Autodesk Inventor part; units mm, degrees
(part 11 of 13)
  spline S1517 degree 3 poles (37.29, 16.1547) (37.0431, 16.1547) (36.843, 15.9546) (36.843, 15.7078) knots 0 0 0 0 1 1 1 1
  line L4777 (37.29, 16.1547) -> (37.0431, 16.1547) construction
  line L4778 (37.0431, 16.1547) -> (36.843, 15.9546) construction
  line L4779 (36.843, 15.9546) -> (36.843, 15.7078) construction
  spline S1518 degree 3 poles (36.843, 15.7078) (36.843, 15.461) (37.0431, 15.2608) (37.29, 15.2608) knots 0 0 0 0 1 1 1 1
  line L4780 (36.843, 15.7078) -> (36.843, 15.461) construction
  line L4781 (36.843, 15.461) -> (37.0431, 15.2608) construction
  line L4782 (37.0431, 15.2608) -> (37.29, 15.2608) construction
  spline S1519 degree 3 poles (37.29, 15.2608) (37.5369, 15.2608) (37.737, 15.461) (37.737, 15.7078) knots 0 0 0 0 1 1 1 1
  line L4783 (37.29, 15.2608) -> (37.5369, 15.2608) construction
  line L4784 (37.5369, 15.2608) -> (37.737, 15.461) construction
  line L4785 (37.737, 15.461) -> (37.737, 15.7078) construction
  spline S1520 degree 3 poles (35.1829, 18.2619) (35.1829, 18.5087) (34.9826, 18.7088) (34.7358, 18.7088) knots 0 0 0 0 1 1 1 1
  line L4786 (35.1829, 18.2619) -> (35.1829, 18.5087) construction
  line L4787 (35.1829, 18.5087) -> (34.9826, 18.7088) construction
  line L4788 (34.9826, 18.7088) -> (34.7358, 18.7088) construction
  spline S1521 degree 3 poles (34.7358, 18.7088) (34.4891, 18.7088) (34.289, 18.5087) (34.289, 18.2619) knots 0 0 0 0 1 1 1 1
  line L4789 (34.7358, 18.7088) -> (34.4891, 18.7088) construction
  line L4790 (34.4891, 18.7088) -> (34.289, 18.5087) construction
  line L4791 (34.289, 18.5087) -> (34.289, 18.2619) construction
  spline S1522 degree 3 poles (34.289, 18.2619) (34.289, 18.0151) (34.4891, 17.8149) (34.7358, 17.8149) knots 0 0 0 0 1 1 1 1
  line L4792 (34.289, 18.2619) -> (34.289, 18.0151) construction
  line L4793 (34.289, 18.0151) -> (34.4891, 17.8149) construction
  line L4794 (34.4891, 17.8149) -> (34.7358, 17.8149) construction
  spline S1523 degree 3 poles (34.7358, 17.8149) (34.9826, 17.8149) (35.1829, 18.0151) (35.1829, 18.2619) knots 0 0 0 0 1 1 1 1
  line L4795 (34.7358, 17.8149) -> (34.9826, 17.8149) construction
  line L4796 (34.9826, 17.8149) -> (35.1829, 18.0151) construction
  line L4797 (35.1829, 18.0151) -> (35.1829, 18.2619) construction
  spline S1524 degree 3 poles (37.737, 18.2619) (37.737, 18.5087) (37.5369, 18.7088) (37.29, 18.7088) knots 0 0 0 0 1 1 1 1
  line L4798 (37.737, 18.2619) -> (37.737, 18.5087) construction
  line L4799 (37.737, 18.5087) -> (37.5369, 18.7088) construction
  line L4800 (37.5369, 18.7088) -> (37.29, 18.7088) construction
  spline S1525 degree 3 poles (37.29, 18.7088) (37.0431, 18.7088) (36.843, 18.5087) (36.843, 18.2619) knots 0 0 0 0 1 1 1 1
  line L4801 (37.29, 18.7088) -> (37.0431, 18.7088) construction
  line L4802 (37.0431, 18.7088) -> (36.843, 18.5087) construction
  line L4803 (36.843, 18.5087) -> (36.843, 18.2619) construction
  spline S1526 degree 3 poles (36.843, 18.2619) (36.843, 18.0151) (37.0431, 17.8149) (37.29, 17.8149) knots 0 0 0 0 1 1 1 1
  line L4804 (36.843, 18.2619) -> (36.843, 18.0151) construction
  line L4805 (36.843, 18.0151) -> (37.0431, 17.8149) construction
  line L4806 (37.0431, 17.8149) -> (37.29, 17.8149) construction
  spline S1527 degree 3 poles (37.29, 17.8149) (37.5369, 17.8149) (37.737, 18.0151) (37.737, 18.2619) knots 0 0 0 0 1 1 1 1
  line L4807 (37.29, 17.8149) -> (37.5369, 17.8149) construction
  line L4808 (37.5369, 17.8149) -> (37.737, 18.0151) construction
  line L4809 (37.737, 18.0151) -> (37.737, 18.2619) construction
  spline S1528 degree 3 poles (35.1829, 20.816) (35.1829, 21.0628) (34.9826, 21.2629) (34.7358, 21.2629) knots 0 0 0 0 1 1 1 1
  line L4810 (35.1829, 20.816) -> (35.1829, 21.0628) construction
  line L4811 (35.1829, 21.0628) -> (34.9826, 21.2629) construction
  line L4812 (34.9826, 21.2629) -> (34.7358, 21.2629) construction
  spline S1529 degree 3 poles (34.7358, 21.2629) (34.4891, 21.2629) (34.289, 21.0628) (34.289, 20.816) knots 0 0 0 0 1 1 1 1
  line L4813 (34.7358, 21.2629) -> (34.4891, 21.2629) construction
  line L4814 (34.4891, 21.2629) -> (34.289, 21.0628) construction
  line L4815 (34.289, 21.0628) -> (34.289, 20.816) construction
  spline S1530 degree 3 poles (34.289, 20.816) (34.289, 20.5692) (34.4891, 20.369) (34.7358, 20.369) knots 0 0 0 0 1 1 1 1
  line L4816 (34.289, 20.816) -> (34.289, 20.5692) construction
  line L4817 (34.289, 20.5692) -> (34.4891, 20.369) construction
  line L4818 (34.4891, 20.369) -> (34.7358, 20.369) construction
  spline S1531 degree 3 poles (34.7358, 20.369) (34.9826, 20.369) (35.1829, 20.5692) (35.1829, 20.816) knots 0 0 0 0 1 1 1 1
  line L4819 (34.7358, 20.369) -> (34.9826, 20.369) construction
  line L4820 (34.9826, 20.369) -> (35.1829, 20.5692) construction
  line L4821 (35.1829, 20.5692) -> (35.1829, 20.816) construction
  spline S1532 degree 3 poles (35.1829, 23.3701) (35.1829, 23.6169) (34.9826, 23.817) (34.7358, 23.817) knots 0 0 0 0 1 1 1 1
  line L4822 (35.1829, 23.3701) -> (35.1829, 23.6169) construction
  line L4823 (35.1829, 23.6169) -> (34.9826, 23.817) construction
  line L4824 (34.9826, 23.817) -> (34.7358, 23.817) construction
  spline S1533 degree 3 poles (34.7358, 23.817) (34.4891, 23.817) (34.289, 23.6169) (34.289, 23.3701) knots 0 0 0 0 1 1 1 1
  line L4825 (34.7358, 23.817) -> (34.4891, 23.817) construction
  line L4826 (34.4891, 23.817) -> (34.289, 23.6169) construction
  line L4827 (34.289, 23.6169) -> (34.289, 23.3701) construction
  spline S1534 degree 3 poles (34.289, 23.3701) (34.289, 23.1233) (34.4891, 22.9231) (34.7358, 22.9231) knots 0 0 0 0 1 1 1 1
  line L4828 (34.289, 23.3701) -> (34.289, 23.1233) construction
  line L4829 (34.289, 23.1233) -> (34.4891, 22.9231) construction
  line L4830 (34.4891, 22.9231) -> (34.7358, 22.9231) construction
  spline S1535 degree 3 poles (34.7358, 22.9231) (34.9826, 22.9231) (35.1829, 23.1233) (35.1829, 23.3701) knots 0 0 0 0 1 1 1 1
  line L4831 (34.7358, 22.9231) -> (34.9826, 22.9231) construction
  line L4832 (34.9826, 22.9231) -> (35.1829, 23.1233) construction
  line L4833 (35.1829, 23.1233) -> (35.1829, 23.3701) construction
  spline S1536 degree 3 poles (35.1829, 25.9242) (35.1829, 26.171) (34.9826, 26.3711) (34.7358, 26.3711) knots 0 0 0 0 1 1 1 1
  line L4834 (35.1829, 25.9242) -> (35.1829, 26.171) construction
  line L4835 (35.1829, 26.171) -> (34.9826, 26.3711) construction
  line L4836 (34.9826, 26.3711) -> (34.7358, 26.3711) construction
  spline S1537 degree 3 poles (34.7358, 26.3711) (34.4891, 26.3711) (34.289, 26.171) (34.289, 25.9242) knots 0 0 0 0 1 1 1 1
  line L4837 (34.7358, 26.3711) -> (34.4891, 26.3711) construction
  line L4838 (34.4891, 26.3711) -> (34.289, 26.171) construction
  line L4839 (34.289, 26.171) -> (34.289, 25.9242) construction
  spline S1538 degree 3 poles (34.289, 25.9242) (34.289, 25.6775) (34.4891, 25.4772) (34.7358, 25.4772) knots 0 0 0 0 1 1 1 1
  line L4840 (34.289, 25.9242) -> (34.289, 25.6775) construction
  line L4841 (34.289, 25.6775) -> (34.4891, 25.4772) construction
  line L4842 (34.4891, 25.4772) -> (34.7358, 25.4772) construction
  spline S1539 degree 3 poles (34.7358, 25.4772) (34.9826, 25.4772) (35.1829, 25.6775) (35.1829, 25.9242) knots 0 0 0 0 1 1 1 1
  line L4843 (34.7358, 25.4772) -> (34.9826, 25.4772) construction
  line L4844 (34.9826, 25.4772) -> (35.1829, 25.6775) construction
  line L4845 (35.1829, 25.6775) -> (35.1829, 25.9242) construction
  spline S1540 degree 3 poles (35.1829, 28.4784) (35.1829, 28.7251) (34.9826, 28.9252) (34.7358, 28.9252) knots 0 0 0 0 1 1 1 1
  line L4846 (35.1829, 28.4784) -> (35.1829, 28.7251) construction
  line L4847 (35.1829, 28.7251) -> (34.9826, 28.9252) construction
  line L4848 (34.9826, 28.9252) -> (34.7358, 28.9252) construction
  spline S1541 degree 3 poles (34.7358, 28.9252) (34.4891, 28.9252) (34.289, 28.7251) (34.289, 28.4784) knots 0 0 0 0 1 1 1 1
  line L4849 (34.7358, 28.9252) -> (34.4891, 28.9252) construction
  line L4850 (34.4891, 28.9252) -> (34.289, 28.7251) construction
  line L4851 (34.289, 28.7251) -> (34.289, 28.4784) construction
  spline S1542 degree 3 poles (34.289, 28.4784) (34.289, 28.2316) (34.4891, 28.0313) (34.7358, 28.0313) knots 0 0 0 0 1 1 1 1
  line L4852 (34.289, 28.4784) -> (34.289, 28.2316) construction
  line L4853 (34.289, 28.2316) -> (34.4891, 28.0313) construction
  line L4854 (34.4891, 28.0313) -> (34.7358, 28.0313) construction
  spline S1543 degree 3 poles (34.7358, 28.0313) (34.9826, 28.0313) (35.1829, 28.2316) (35.1829, 28.4784) knots 0 0 0 0 1 1 1 1
  line L4855 (34.7358, 28.0313) -> (34.9826, 28.0313) construction
  line L4856 (34.9826, 28.0313) -> (35.1829, 28.2316) construction
  line L4857 (35.1829, 28.2316) -> (35.1829, 28.4784) construction
  spline S1544 degree 3 poles (35.1829, 31.0325) (35.1829, 31.2793) (34.9826, 31.4793) (34.7358, 31.4793) knots 0 0 0 0 1 1 1 1
  line L4858 (35.1829, 31.0325) -> (35.1829, 31.2793) construction
  line L4859 (35.1829, 31.2793) -> (34.9826, 31.4793) construction
  line L4860 (34.9826, 31.4793) -> (34.7358, 31.4793) construction
  spline S1545 degree 3 poles (34.7358, 31.4793) (34.4891, 31.4793) (34.289, 31.2793) (34.289, 31.0325) knots 0 0 0 0 1 1 1 1
  line L4861 (34.7358, 31.4793) -> (34.4891, 31.4793) construction
  line L4862 (34.4891, 31.4793) -> (34.289, 31.2793) construction
  line L4863 (34.289, 31.2793) -> (34.289, 31.0325) construction
  spline S1546 degree 3 poles (34.289, 31.0325) (34.289, 30.7857) (34.4891, 30.5854) (34.7358, 30.5854) knots 0 0 0 0 1 1 1 1
  line L4864 (34.289, 31.0325) -> (34.289, 30.7857) construction
  line L4865 (34.289, 30.7857) -> (34.4891, 30.5854) construction
  line L4866 (34.4891, 30.5854) -> (34.7358, 30.5854) construction
  spline S1547 degree 3 poles (34.7358, 30.5854) (34.9826, 30.5854) (35.1829, 30.7857) (35.1829, 31.0325) knots 0 0 0 0 1 1 1 1
  line L4867 (34.7358, 30.5854) -> (34.9826, 30.5854) construction
  line L4868 (34.9826, 30.5854) -> (35.1829, 30.7857) construction
  line L4869 (35.1829, 30.7857) -> (35.1829, 31.0325) construction
  spline S1548 degree 3 poles (37.737, 20.816) (37.737, 21.0628) (37.5369, 21.2629) (37.29, 21.2629) knots 0 0 0 0 1 1 1 1
  line L4870 (37.737, 20.816) -> (37.737, 21.0628) construction
  line L4871 (37.737, 21.0628) -> (37.5369, 21.2629) construction
  line L4872 (37.5369, 21.2629) -> (37.29, 21.2629) construction
  spline S1549 degree 3 poles (37.29, 21.2629) (37.0431, 21.2629) (36.843, 21.0628) (36.843, 20.816) knots 0 0 0 0 1 1 1 1
  line L4873 (37.29, 21.2629) -> (37.0431, 21.2629) construction
  line L4874 (37.0431, 21.2629) -> (36.843, 21.0628) construction
  line L4875 (36.843, 21.0628) -> (36.843, 20.816) construction
  spline S1550 degree 3 poles (36.843, 20.816) (36.843, 20.5692) (37.0431, 20.369) (37.29, 20.369) knots 0 0 0 0 1 1 1 1
  line L4876 (36.843, 20.816) -> (36.843, 20.5692) construction
  line L4877 (36.843, 20.5692) -> (37.0431, 20.369) construction
  line L4878 (37.0431, 20.369) -> (37.29, 20.369) construction
  spline S1551 degree 3 poles (37.29, 20.369) (37.5369, 20.369) (37.737, 20.5692) (37.737, 20.816) knots 0 0 0 0 1 1 1 1
  line L4879 (37.29, 20.369) -> (37.5369, 20.369) construction
  line L4880 (37.5369, 20.369) -> (37.737, 20.5692) construction
  line L4881 (37.737, 20.5692) -> (37.737, 20.816) construction
  spline S1552 degree 3 poles (37.737, 23.3701) (37.737, 23.6169) (37.5369, 23.817) (37.29, 23.817) knots 0 0 0 0 1 1 1 1
  line L4882 (37.737, 23.3701) -> (37.737, 23.6169) construction
  line L4883 (37.737, 23.6169) -> (37.5369, 23.817) construction
  line L4884 (37.5369, 23.817) -> (37.29, 23.817) construction
  spline S1553 degree 3 poles (37.29, 23.817) (37.0431, 23.817) (36.843, 23.6169) (36.843, 23.3701) knots 0 0 0 0 1 1 1 1
  line L4885 (37.29, 23.817) -> (37.0431, 23.817) construction
  line L4886 (37.0431, 23.817) -> (36.843, 23.6169) construction
  line L4887 (36.843, 23.6169) -> (36.843, 23.3701) construction
  spline S1554 degree 3 poles (36.843, 23.3701) (36.843, 23.1233) (37.0431, 22.9231) (37.29, 22.9231) knots 0 0 0 0 1 1 1 1
  line L4888 (36.843, 23.3701) -> (36.843, 23.1233) construction
  line L4889 (36.843, 23.1233) -> (37.0431, 22.9231) construction
  line L4890 (37.0431, 22.9231) -> (37.29, 22.9231) construction
  spline S1555 degree 3 poles (37.29, 22.9231) (37.5369, 22.9231) (37.737, 23.1233) (37.737, 23.3701) knots 0 0 0 0 1 1 1 1
  line L4891 (37.29, 22.9231) -> (37.5369, 22.9231) construction
  line L4892 (37.5369, 22.9231) -> (37.737, 23.1233) construction
  line L4893 (37.737, 23.1233) -> (37.737, 23.3701) construction
  spline S1556 degree 3 poles (37.737, 25.9242) (37.737, 26.171) (37.5369, 26.3711) (37.29, 26.3711) knots 0 0 0 0 1 1 1 1
  line L4894 (37.737, 25.9242) -> (37.737, 26.171) construction
  line L4895 (37.737, 26.171) -> (37.5369, 26.3711) construction
  line L4896 (37.5369, 26.3711) -> (37.29, 26.3711) construction
  spline S1557 degree 3 poles (37.29, 26.3711) (37.0431, 26.3711) (36.843, 26.171) (36.843, 25.9242) knots 0 0 0 0 1 1 1 1
  line L4897 (37.29, 26.3711) -> (37.0431, 26.3711) construction
  line L4898 (37.0431, 26.3711) -> (36.843, 26.171) construction
  line L4899 (36.843, 26.171) -> (36.843, 25.9242) construction
  spline S1558 degree 3 poles (36.843, 25.9242) (36.843, 25.6775) (37.0431, 25.4772) (37.29, 25.4772) knots 0 0 0 0 1 1 1 1
  line L4900 (36.843, 25.9242) -> (36.843, 25.6775) construction
  line L4901 (36.843, 25.6775) -> (37.0431, 25.4772) construction
  line L4902 (37.0431, 25.4772) -> (37.29, 25.4772) construction
  spline S1559 degree 3 poles (37.29, 25.4772) (37.5369, 25.4772) (37.737, 25.6775) (37.737, 25.9242) knots 0 0 0 0 1 1 1 1
  line L4903 (37.29, 25.4772) -> (37.5369, 25.4772) construction
  line L4904 (37.5369, 25.4772) -> (37.737, 25.6775) construction
  line L4905 (37.737, 25.6775) -> (37.737, 25.9242) construction
  spline S1560 degree 3 poles (37.737, 28.4784) (37.737, 28.7251) (37.5369, 28.9252) (37.29, 28.9252) knots 0 0 0 0 1 1 1 1
  line L4906 (37.737, 28.4784) -> (37.737, 28.7251) construction
  line L4907 (37.737, 28.7251) -> (37.5369, 28.9252) construction
  line L4908 (37.5369, 28.9252) -> (37.29, 28.9252) construction
  spline S1561 degree 3 poles (37.29, 28.9252) (37.0431, 28.9252) (36.843, 28.7251) (36.843, 28.4784) knots 0 0 0 0 1 1 1 1
  line L4909 (37.29, 28.9252) -> (37.0431, 28.9252) construction
  line L4910 (37.0431, 28.9252) -> (36.843, 28.7251) construction
  line L4911 (36.843, 28.7251) -> (36.843, 28.4784) construction
  spline S1562 degree 3 poles (36.843, 28.4784) (36.843, 28.2316) (37.0431, 28.0313) (37.29, 28.0313) knots 0 0 0 0 1 1 1 1
  line L4912 (36.843, 28.4784) -> (36.843, 28.2316) construction
  line L4913 (36.843, 28.2316) -> (37.0431, 28.0313) construction
  line L4914 (37.0431, 28.0313) -> (37.29, 28.0313) construction
  spline S1563 degree 3 poles (37.29, 28.0313) (37.5369, 28.0313) (37.737, 28.2316) (37.737, 28.4784) knots 0 0 0 0 1 1 1 1
  line L4915 (37.29, 28.0313) -> (37.5369, 28.0313) construction
  line L4916 (37.5369, 28.0313) -> (37.737, 28.2316) construction
  line L4917 (37.737, 28.2316) -> (37.737, 28.4784) construction
  spline S1564 degree 3 poles (37.737, 31.0325) (37.737, 31.2793) (37.5369, 31.4793) (37.29, 31.4793) knots 0 0 0 0 1 1 1 1
  line L4918 (37.737, 31.0325) -> (37.737, 31.2793) construction
  line L4919 (37.737, 31.2793) -> (37.5369, 31.4793) construction
  line L4920 (37.5369, 31.4793) -> (37.29, 31.4793) construction
  spline S1565 degree 3 poles (37.29, 31.4793) (37.0431, 31.4793) (36.843, 31.2793) (36.843, 31.0325) knots 0 0 0 0 1 1 1 1
  line L4921 (37.29, 31.4793) -> (37.0431, 31.4793) construction
  line L4922 (37.0431, 31.4793) -> (36.843, 31.2793) construction
  line L4923 (36.843, 31.2793) -> (36.843, 31.0325) construction
  spline S1566 degree 3 poles (36.843, 31.0325) (36.843, 30.7857) (37.0431, 30.5854) (37.29, 30.5854) knots 0 0 0 0 1 1 1 1
  line L4924 (36.843, 31.0325) -> (36.843, 30.7857) construction
  line L4925 (36.843, 30.7857) -> (37.0431, 30.5854) construction
  line L4926 (37.0431, 30.5854) -> (37.29, 30.5854) construction
  spline S1567 degree 3 poles (37.29, 30.5854) (37.5369, 30.5854) (37.737, 30.7857) (37.737, 31.0325) knots 0 0 0 0 1 1 1 1
  line L4927 (37.29, 30.5854) -> (37.5369, 30.5854) construction
  line L4928 (37.5369, 30.5854) -> (37.737, 30.7857) construction
  line L4929 (37.737, 30.7857) -> (37.737, 31.0325) construction
  spline S1568 degree 3 poles (45.3993, 0.3832) (45.3993, 0.6299) (45.1992, 0.83) (44.9523, 0.83) knots 0 0 0 0 1 1 1 1
  line L4930 (45.3993, 0.3832) -> (45.3993, 0.6299) construction
  line L4931 (45.3993, 0.6299) -> (45.1992, 0.83) construction
  line L4932 (45.1992, 0.83) -> (44.9523, 0.83) construction
  spline S1569 degree 3 poles (44.9523, 0.83) (44.7054, 0.83) (44.5054, 0.6299) (44.5054, 0.3832) knots 0 0 0 0 1 1 1 1
  line L4933 (44.9523, 0.83) -> (44.7054, 0.83) construction
  line L4934 (44.7054, 0.83) -> (44.5054, 0.6299) construction
  line L4935 (44.5054, 0.6299) -> (44.5054, 0.3832) construction
  spline S1570 degree 3 poles (44.5054, 0.3832) (44.5054, 0.1364) (44.7054, -0.0639) (44.9523, -0.0639) knots 0 0 0 0 1 1 1 1
  line L4936 (44.5054, 0.3832) -> (44.5054, 0.1364) construction
  line L4937 (44.5054, 0.1364) -> (44.7054, -0.0639) construction
  line L4938 (44.7054, -0.0639) -> (44.9523, -0.0639) construction
  spline S1571 degree 3 poles (44.9523, -0.0639) (45.1992, -0.0639) (45.3993, 0.1364) (45.3993, 0.3832) knots 0 0 0 0 1 1 1 1
  line L4939 (44.9523, -0.0639) -> (45.1992, -0.0639) construction
  line L4940 (45.1992, -0.0639) -> (45.3993, 0.1364) construction
  line L4941 (45.3993, 0.1364) -> (45.3993, 0.3832) construction
  spline S1572 degree 3 poles (47.9534, 0.3832) (47.9534, 0.6299) (47.7533, 0.83) (47.5064, 0.83) knots 0 0 0 0 1 1 1 1
  line L4942 (47.9534, 0.3832) -> (47.9534, 0.6299) construction
  line L4943 (47.9534, 0.6299) -> (47.7533, 0.83) construction
  line L4944 (47.7533, 0.83) -> (47.5064, 0.83) construction
  spline S1573 degree 3 poles (47.5064, 0.83) (47.2595, 0.83) (47.0595, 0.6299) (47.0595, 0.3832) knots 0 0 0 0 1 1 1 1
  line L4945 (47.5064, 0.83) -> (47.2595, 0.83) construction
  line L4946 (47.2595, 0.83) -> (47.0595, 0.6299) construction
  line L4947 (47.0595, 0.6299) -> (47.0595, 0.3832) construction
  spline S1574 degree 3 poles (47.0595, 0.3832) (47.0595, 0.1364) (47.2595, -0.0639) (47.5064, -0.0639) knots 0 0 0 0 1 1 1 1
  line L4948 (47.0595, 0.3832) -> (47.0595, 0.1364) construction
  line L4949 (47.0595, 0.1364) -> (47.2595, -0.0639) construction
  line L4950 (47.2595, -0.0639) -> (47.5064, -0.0639) construction
  spline S1575 degree 3 poles (47.5064, -0.0639) (47.7533, -0.0639) (47.9534, 0.1364) (47.9534, 0.3832) knots 0 0 0 0 1 1 1 1
  line L4951 (47.5064, -0.0639) -> (47.7533, -0.0639) construction
  line L4952 (47.7533, -0.0639) -> (47.9534, 0.1364) construction
  line L4953 (47.9534, 0.1364) -> (47.9534, 0.3832) construction
  spline S1576 degree 3 poles (46.6763, 9.7057) (46.6763, 10.5872) (45.9615, 11.302) (45.08, 11.302) knots 0 0 0 0 1 1 1 1
  line L4954 (46.6763, 9.7057) -> (46.6763, 10.5872) construction
  line L4955 (46.6763, 10.5872) -> (45.9615, 11.302) construction
  line L4956 (45.9615, 11.302) -> (45.08, 11.302) construction
  spline S1577 degree 3 poles (45.08, 11.302) (44.1985, 11.302) (43.4837, 10.5872) (43.4837, 9.7057) knots 0 0 0 0 1 1 1 1
  line L4957 (45.08, 11.302) -> (44.1985, 11.302) construction
  line L4958 (44.1985, 11.302) -> (43.4837, 10.5872) construction
  line L4959 (43.4837, 10.5872) -> (43.4837, 9.7057) construction
  spline S1578 degree 3 poles (43.4837, 9.7057) (43.4837, 8.8241) (44.1985, 8.1094) (45.08, 8.1094) knots 0 0 0 0 1 1 1 1
  line L4960 (43.4837, 9.7057) -> (43.4837, 8.8241) construction
  line L4961 (43.4837, 8.8241) -> (44.1985, 8.1094) construction
  line L4962 (44.1985, 8.1094) -> (45.08, 8.1094) construction
  spline S1579 degree 3 poles (45.08, 8.1094) (45.9615, 8.1094) (46.6763, 8.8241) (46.6763, 9.7057) knots 0 0 0 0 1 1 1 1
  line L4963 (45.08, 8.1094) -> (45.9615, 8.1094) construction
  line L4964 (45.9615, 8.1094) -> (46.6763, 8.8241) construction
  line L4965 (46.6763, 8.8241) -> (46.6763, 9.7057) construction
  spline S1580 degree 3 poles (52.8701, 9.7057) (52.8701, 10.4814) (52.2411, 11.1103) (51.4653, 11.1103) knots 0 0 0 0 1 1 1 1
  line L4966 (52.8701, 9.7057) -> (52.8701, 10.4814) construction
  line L4967 (52.8701, 10.4814) -> (52.2411, 11.1103) construction
  line L4968 (52.2411, 11.1103) -> (51.4653, 11.1103) construction
  spline S1581 degree 3 poles (51.4653, 11.1103) (50.6895, 11.1103) (50.0605, 10.4814) (50.0605, 9.7057) knots 0 0 0 0 1 1 1 1
  line L4969 (51.4653, 11.1103) -> (50.6895, 11.1103) construction
  line L4970 (50.6895, 11.1103) -> (50.0605, 10.4814) construction
  line L4971 (50.0605, 10.4814) -> (50.0605, 9.7057) construction
  spline S1582 degree 3 poles (50.0605, 9.7057) (50.0605, 8.9299) (50.6895, 8.3009) (51.4653, 8.3009) knots 0 0 0 0 1 1 1 1
  line L4972 (50.0605, 9.7057) -> (50.0605, 8.9299) construction
  line L4973 (50.0605, 8.9299) -> (50.6895, 8.3009) construction
  line L4974 (50.6895, 8.3009) -> (51.4653, 8.3009) construction
  spline S1583 degree 3 poles (51.4653, 8.3009) (52.2411, 8.3009) (52.8701, 8.9299) (52.8701, 9.7057) knots 0 0 0 0 1 1 1 1
  line L4975 (51.4653, 8.3009) -> (52.2411, 8.3009) construction
  line L4976 (52.2411, 8.3009) -> (52.8701, 8.9299) construction
  line L4977 (52.8701, 8.9299) -> (52.8701, 9.7057) construction
  spline S1584 degree 3 poles (49.6774, 14.303) (49.6774, 15.0787) (49.0485, 15.7078) (48.2727, 15.7078) knots 0 0 0 0 1 1 1 1
  line L4978 (49.6774, 14.303) -> (49.6774, 15.0787) construction
  line L4979 (49.6774, 15.0787) -> (49.0485, 15.7078) construction
  line L4980 (49.0485, 15.7078) -> (48.2727, 15.7078) construction
  spline S1585 degree 3 poles (48.2727, 15.7078) (47.4969, 15.7078) (46.8679, 15.0787) (46.8679, 14.303) knots 0 0 0 0 1 1 1 1
  line L4981 (48.2727, 15.7078) -> (47.4969, 15.7078) construction
  line L4982 (47.4969, 15.7078) -> (46.8679, 15.0787) construction
  line L4983 (46.8679, 15.0787) -> (46.8679, 14.303) construction
  spline S1586 degree 3 poles (46.8679, 14.303) (46.8679, 13.5273) (47.4969, 12.8983) (48.2727, 12.8983) knots 0 0 0 0 1 1 1 1
  line L4984 (46.8679, 14.303) -> (46.8679, 13.5273) construction
  line L4985 (46.8679, 13.5273) -> (47.4969, 12.8983) construction
  line L4986 (47.4969, 12.8983) -> (48.2727, 12.8983) construction
  spline S1587 degree 3 poles (48.2727, 12.8983) (49.0485, 12.8983) (49.6774, 13.5273) (49.6774, 14.303) knots 0 0 0 0 1 1 1 1
  line L4987 (48.2727, 12.8983) -> (49.0485, 12.8983) construction
  line L4988 (49.0485, 12.8983) -> (49.6774, 13.5273) construction
  line L4989 (49.6774, 13.5273) -> (49.6774, 14.303) construction
  spline S1588 degree 3 poles (9.6418, 0.3832) (9.6418, 0.6299) (9.4415, 0.83) (9.1948, 0.83) knots 0 0 0 0 1 1 1 1
  line L4990 (9.6418, 0.3832) -> (9.6418, 0.6299) construction
  line L4991 (9.6418, 0.6299) -> (9.4415, 0.83) construction
  line L4992 (9.4415, 0.83) -> (9.1948, 0.83) construction
  spline S1589 degree 3 poles (9.1948, 0.83) (8.948, 0.83) (8.7479, 0.6299) (8.7479, 0.3832) knots 0 0 0 0 1 1 1 1
  line L4993 (9.1948, 0.83) -> (8.948, 0.83) construction
  line L4994 (8.948, 0.83) -> (8.7479, 0.6299) construction
  line L4995 (8.7479, 0.6299) -> (8.7479, 0.3832) construction
  spline S1590 degree 3 poles (8.7479, 0.3832) (8.7479, 0.1364) (8.948, -0.0639) (9.1948, -0.0639) knots 0 0 0 0 1 1 1 1
  line L4996 (8.7479, 0.3832) -> (8.7479, 0.1364) construction
  line L4997 (8.7479, 0.1364) -> (8.948, -0.0639) construction
  line L4998 (8.948, -0.0639) -> (9.1948, -0.0639) construction
  spline S1591 degree 3 poles (9.1948, -0.0639) (9.4415, -0.0639) (9.6418, 0.1364) (9.6418, 0.3832) knots 0 0 0 0 1 1 1 1
  line L4999 (9.1948, -0.0639) -> (9.4415, -0.0639) construction
  line L5000 (9.4415, -0.0639) -> (9.6418, 0.1364) construction
  line L5001 (9.6418, 0.1364) -> (9.6418, 0.3832) construction
  spline S1592 degree 3 poles (12.1959, 0.3832) (12.1959, 0.6299) (11.9957, 0.83) (11.7489, 0.83) knots 0 0 0 0 1 1 1 1
  line L5002 (12.1959, 0.3832) -> (12.1959, 0.6299) construction
  line L5003 (12.1959, 0.6299) -> (11.9957, 0.83) construction
  line L5004 (11.9957, 0.83) -> (11.7489, 0.83) construction
  spline S1593 degree 3 poles (11.7489, 0.83) (11.5021, 0.83) (11.302, 0.6299) (11.302, 0.3832) knots 0 0 0 0 1 1 1 1
  line L5005 (11.7489, 0.83) -> (11.5021, 0.83) construction
  line L5006 (11.5021, 0.83) -> (11.302, 0.6299) construction
  line L5007 (11.302, 0.6299) -> (11.302, 0.3832) construction
  spline S1594 degree 3 poles (11.302, 0.3832) (11.302, 0.1364) (11.5021, -0.0639) (11.7489, -0.0639) knots 0 0 0 0 1 1 1 1
  line L5008 (11.302, 0.3832) -> (11.302, 0.1364) construction
  line L5009 (11.302, 0.1364) -> (11.5021, -0.0639) construction
  line L5010 (11.5021, -0.0639) -> (11.7489, -0.0639) construction
  spline S1595 degree 3 poles (11.7489, -0.0639) (11.9957, -0.0639) (12.1959, 0.1364) (12.1959, 0.3832) knots 0 0 0 0 1 1 1 1
  line L5011 (11.7489, -0.0639) -> (11.9957, -0.0639) construction
  line L5012 (11.9957, -0.0639) -> (12.1959, 0.1364) construction
  line L5013 (12.1959, 0.1364) -> (12.1959, 0.3832) construction
  spline S1596 degree 3 poles (14.75, 0.3832) (14.75, 0.6299) (14.5498, 0.83) (14.303, 0.83) knots 0 0 0 0 1 1 1 1
  line L5014 (14.75, 0.3832) -> (14.75, 0.6299) construction
  line L5015 (14.75, 0.6299) -> (14.5498, 0.83) construction
  line L5016 (14.5498, 0.83) -> (14.303, 0.83) construction
  spline S1597 degree 3 poles (14.303, 0.83) (14.0562, 0.83) (13.8561, 0.6299) (13.8561, 0.3832) knots 0 0 0 0 1 1 1 1
  line L5017 (14.303, 0.83) -> (14.0562, 0.83) construction
  line L5018 (14.0562, 0.83) -> (13.8561, 0.6299) construction
  line L5019 (13.8561, 0.6299) -> (13.8561, 0.3832) construction
  spline S1598 degree 3 poles (13.8561, 0.3832) (13.8561, 0.1364) (14.0562, -0.0639) (14.303, -0.0639) knots 0 0 0 0 1 1 1 1
  line L5020 (13.8561, 0.3832) -> (13.8561, 0.1364) construction
  line L5021 (13.8561, 0.1364) -> (14.0562, -0.0639) construction
  line L5022 (14.0562, -0.0639) -> (14.303, -0.0639) construction
  spline S1599 degree 3 poles (14.303, -0.0639) (14.5498, -0.0639) (14.75, 0.1364) (14.75, 0.3832) knots 0 0 0 0 1 1 1 1
  line L5023 (14.303, -0.0639) -> (14.5498, -0.0639) construction
  line L5024 (14.5498, -0.0639) -> (14.75, 0.1364) construction
  line L5025 (14.75, 0.1364) -> (14.75, 0.3832) construction
  spline S1600 degree 3 poles (17.3041, 0.3832) (17.3041, 0.6299) (17.1039, 0.83) (16.8571, 0.83) knots 0 0 0 0 1 1 1 1
  line L5026 (17.3041, 0.3832) -> (17.3041, 0.6299) construction
  line L5027 (17.3041, 0.6299) -> (17.1039, 0.83) construction
  line L5028 (17.1039, 0.83) -> (16.8571, 0.83) construction
  spline S1601 degree 3 poles (16.8571, 0.83) (16.6103, 0.83) (16.4102, 0.6299) (16.4102, 0.3832) knots 0 0 0 0 1 1 1 1
  line L5029 (16.8571, 0.83) -> (16.6103, 0.83) construction
  line L5030 (16.6103, 0.83) -> (16.4102, 0.6299) construction
  line L5031 (16.4102, 0.6299) -> (16.4102, 0.3832) construction
  spline S1602 degree 3 poles (16.4102, 0.3832) (16.4102, 0.1364) (16.6103, -0.0639) (16.8571, -0.0639) knots 0 0 0 0 1 1 1 1
  line L5032 (16.4102, 0.3832) -> (16.4102, 0.1364) construction
  line L5033 (16.4102, 0.1364) -> (16.6103, -0.0639) construction
  line L5034 (16.6103, -0.0639) -> (16.8571, -0.0639) construction
  spline S1603 degree 3 poles (16.8571, -0.0639) (17.1039, -0.0639) (17.3041, 0.1364) (17.3041, 0.3832) knots 0 0 0 0 1 1 1 1
  line L5035 (16.8571, -0.0639) -> (17.1039, -0.0639) construction
  line L5036 (17.1039, -0.0639) -> (17.3041, 0.1364) construction
  line L5037 (17.3041, 0.1364) -> (17.3041, 0.3832) construction
  spline S1604 degree 3 poles (17.3041, 2.9373) (17.3041, 3.1841) (17.1039, 3.3841) (16.8571, 3.3841) knots 0 0 0 0 1 1 1 1
  line L5038 (17.3041, 2.9373) -> (17.3041, 3.1841) construction
  line L5039 (17.3041, 3.1841) -> (17.1039, 3.3841) construction
  line L5040 (17.1039, 3.3841) -> (16.8571, 3.3841) construction
  spline S1605 degree 3 poles (16.8571, 3.3841) (16.6103, 3.3841) (16.4102, 3.1841) (16.4102, 2.9373) knots 0 0 0 0 1 1 1 1
  line L5041 (16.8571, 3.3841) -> (16.6103, 3.3841) construction
  line L5042 (16.6103, 3.3841) -> (16.4102, 3.1841) construction
  line L5043 (16.4102, 3.1841) -> (16.4102, 2.9373) construction
  spline S1606 degree 3 poles (16.4102, 2.9373) (16.4102, 2.6905) (16.6103, 2.4902) (16.8571, 2.4902) knots 0 0 0 0 1 1 1 1
  line L5044 (16.4102, 2.9373) -> (16.4102, 2.6905) construction
  line L5045 (16.4102, 2.6905) -> (16.6103, 2.4902) construction
  line L5046 (16.6103, 2.4902) -> (16.8571, 2.4902) construction
  spline S1607 degree 3 poles (16.8571, 2.4902) (17.1039, 2.4902) (17.3041, 2.6905) (17.3041, 2.9373) knots 0 0 0 0 1 1 1 1
  line L5047 (16.8571, 2.4902) -> (17.1039, 2.4902) construction
  line L5048 (17.1039, 2.4902) -> (17.3041, 2.6905) construction
  line L5049 (17.3041, 2.6905) -> (17.3041, 2.9373) construction
  spline S1608 degree 3 poles (19.8582, 2.9373) (19.8582, 3.1841) (19.658, 3.3841) (19.4112, 3.3841) knots 0 0 0 0 1 1 1 1
  line L5050 (19.8582, 2.9373) -> (19.8582, 3.1841) construction
  line L5051 (19.8582, 3.1841) -> (19.658, 3.3841) construction
  line L5052 (19.658, 3.3841) -> (19.4112, 3.3841) construction
  spline S1609 degree 3 poles (19.4112, 3.3841) (19.1644, 3.3841) (18.9643, 3.1841) (18.9643, 2.9373) knots 0 0 0 0 1 1 1 1
  line L5053 (19.4112, 3.3841) -> (19.1644, 3.3841) construction
  line L5054 (19.1644, 3.3841) -> (18.9643, 3.1841) construction
  line L5055 (18.9643, 3.1841) -> (18.9643, 2.9373) construction
  spline S1610 degree 3 poles (18.9643, 2.9373) (18.9643, 2.6905) (19.1644, 2.4902) (19.4112, 2.4902) knots 0 0 0 0 1 1 1 1
  line L5056 (18.9643, 2.9373) -> (18.9643, 2.6905) construction
  line L5057 (18.9643, 2.6905) -> (19.1644, 2.4902) construction
  line L5058 (19.1644, 2.4902) -> (19.4112, 2.4902) construction
  spline S1611 degree 3 poles (19.4112, 2.4902) (19.658, 2.4902) (19.8582, 2.6905) (19.8582, 2.9373) knots 0 0 0 0 1 1 1 1
  line L5059 (19.4112, 2.4902) -> (19.658, 2.4902) construction
  line L5060 (19.658, 2.4902) -> (19.8582, 2.6905) construction
  line L5061 (19.8582, 2.6905) -> (19.8582, 2.9373) construction
  spline S1612 degree 3 poles (26.2435, 0.3832) (26.2435, 0.6299) (26.0433, 0.83) (25.7965, 0.83) knots 0 0 0 0 1 1 1 1
  line L5062 (26.2435, 0.3832) -> (26.2435, 0.6299) construction
  line L5063 (26.2435, 0.6299) -> (26.0433, 0.83) construction
  line L5064 (26.0433, 0.83) -> (25.7965, 0.83) construction
  spline S1613 degree 3 poles (25.7965, 0.83) (25.5497, 0.83) (25.3496, 0.6299) (25.3496, 0.3832) knots 0 0 0 0 1 1 1 1
  line L5065 (25.7965, 0.83) -> (25.5497, 0.83) construction
  line L5066 (25.5497, 0.83) -> (25.3496, 0.6299) construction
  line L5067 (25.3496, 0.6299) -> (25.3496, 0.3832) construction
  spline S1614 degree 3 poles (25.3496, 0.3832) (25.3496, 0.1364) (25.5497, -0.0639) (25.7965, -0.0639) knots 0 0 0 0 1 1 1 1
  line L5068 (25.3496, 0.3832) -> (25.3496, 0.1364) construction
  line L5069 (25.3496, 0.1364) -> (25.5497, -0.0639) construction
  line L5070 (25.5497, -0.0639) -> (25.7965, -0.0639) construction
  spline S1615 degree 3 poles (25.7965, -0.0639) (26.0433, -0.0639) (26.2435, 0.1364) (26.2435, 0.3832) knots 0 0 0 0 1 1 1 1
  line L5071 (25.7965, -0.0639) -> (26.0433, -0.0639) construction
  line L5072 (26.0433, -0.0639) -> (26.2435, 0.1364) construction
  line L5073 (26.2435, 0.1364) -> (26.2435, 0.3832) construction
  spline S1616 degree 3 poles (23.6894, 0.3832) (23.6894, 0.6299) (23.4891, 0.83) (23.2424, 0.83) knots 0 0 0 0 1 1 1 1
  line L5074 (23.6894, 0.3832) -> (23.6894, 0.6299) construction
  line L5075 (23.6894, 0.6299) -> (23.4891, 0.83) construction
  line L5076 (23.4891, 0.83) -> (23.2424, 0.83) construction
  spline S1617 degree 3 poles (23.2424, 0.83) (22.9956, 0.83) (22.7955, 0.6299) (22.7955, 0.3832) knots 0 0 0 0 1 1 1 1
  line L5077 (23.2424, 0.83) -> (22.9956, 0.83) construction
  line L5078 (22.9956, 0.83) -> (22.7955, 0.6299) construction
  line L5079 (22.7955, 0.6299) -> (22.7955, 0.3832) construction
  spline S1618 degree 3 poles (22.7955, 0.3832) (22.7955, 0.1364) (22.9956, -0.0639) (23.2424, -0.0639) knots 0 0 0 0 1 1 1 1
  line L5080 (22.7955, 0.3832) -> (22.7955, 0.1364) construction
  line L5081 (22.7955, 0.1364) -> (22.9956, -0.0639) construction
  line L5082 (22.9956, -0.0639) -> (23.2424, -0.0639) construction
  spline S1619 degree 3 poles (23.2424, -0.0639) (23.4891, -0.0639) (23.6894, 0.1364) (23.6894, 0.3832) knots 0 0 0 0 1 1 1 1
  line L5083 (23.2424, -0.0639) -> (23.4891, -0.0639) construction
  line L5084 (23.4891, -0.0639) -> (23.6894, 0.1364) construction
  line L5085 (23.6894, 0.1364) -> (23.6894, 0.3832) construction
  spline S1620 degree 3 poles (21.1353, 0.3832) (21.1353, 0.6299) (20.935, 0.83) (20.6882, 0.83) knots 0 0 0 0 1 1 1 1
  line L5086 (21.1353, 0.3832) -> (21.1353, 0.6299) construction
  line L5087 (21.1353, 0.6299) -> (20.935, 0.83) construction
  line L5088 (20.935, 0.83) -> (20.6882, 0.83) construction
  spline S1621 degree 3 poles (20.6882, 0.83) (20.4415, 0.83) (20.2414, 0.6299) (20.2414, 0.3832) knots 0 0 0 0 1 1 1 1
  line L5089 (20.6882, 0.83) -> (20.4415, 0.83) construction
  line L5090 (20.4415, 0.83) -> (20.2414, 0.6299) construction
  line L5091 (20.2414, 0.6299) -> (20.2414, 0.3832) construction
  spline S1622 degree 3 poles (20.2414, 0.3832) (20.2414, 0.1364) (20.4415, -0.0639) (20.6882, -0.0639) knots 0 0 0 0 1 1 1 1
  line L5092 (20.2414, 0.3832) -> (20.2414, 0.1364) construction
  line L5093 (20.2414, 0.1364) -> (20.4415, -0.0639) construction
  line L5094 (20.4415, -0.0639) -> (20.6882, -0.0639) construction
  spline S1623 degree 3 poles (20.6882, -0.0639) (20.935, -0.0639) (21.1353, 0.1364) (21.1353, 0.3832) knots 0 0 0 0 1 1 1 1
  line L5095 (20.6882, -0.0639) -> (20.935, -0.0639) construction
  line L5096 (20.935, -0.0639) -> (21.1353, 0.1364) construction
  line L5097 (21.1353, 0.1364) -> (21.1353, 0.3832) construction
  spline S1624 degree 3 poles (19.8582, 5.4914) (19.8582, 5.7382) (19.658, 5.9382) (19.4112, 5.9382) knots 0 0 0 0 1 1 1 1
  line L5098 (19.8582, 5.4914) -> (19.8582, 5.7382) construction
  line L5099 (19.8582, 5.7382) -> (19.658, 5.9382) construction
  line L5100 (19.658, 5.9382) -> (19.4112, 5.9382) construction
  spline S1625 degree 3 poles (19.4112, 5.9382) (19.1644, 5.9382) (18.9643, 5.7382) (18.9643, 5.4914) knots 0 0 0 0 1 1 1 1
  line L5101 (19.4112, 5.9382) -> (19.1644, 5.9382) construction
  line L5102 (19.1644, 5.9382) -> (18.9643, 5.7382) construction
  line L5103 (18.9643, 5.7382) -> (18.9643, 5.4914) construction
  spline S1626 degree 3 poles (18.9643, 5.4914) (18.9643, 5.2446) (19.1644, 5.0443) (19.4112, 5.0443) knots 0 0 0 0 1 1 1 1
  line L5104 (18.9643, 5.4914) -> (18.9643, 5.2446) construction
  line L5105 (18.9643, 5.2446) -> (19.1644, 5.0443) construction
  line L5106 (19.1644, 5.0443) -> (19.4112, 5.0443) construction
  spline S1627 degree 3 poles (19.4112, 5.0443) (19.658, 5.0443) (19.8582, 5.2446) (19.8582, 5.4914) knots 0 0 0 0 1 1 1 1
  line L5107 (19.4112, 5.0443) -> (19.658, 5.0443) construction
  line L5108 (19.658, 5.0443) -> (19.8582, 5.2446) construction
  line L5109 (19.8582, 5.2446) -> (19.8582, 5.4914) construction
  spline S1628 degree 3 poles (19.8582, 8.0455) (19.8582, 8.2923) (19.658, 8.4923) (19.4112, 8.4923) knots 0 0 0 0 1 1 1 1
  line L5110 (19.8582, 8.0455) -> (19.8582, 8.2923) construction
  line L5111 (19.8582, 8.2923) -> (19.658, 8.4923) construction
  line L5112 (19.658, 8.4923) -> (19.4112, 8.4923) construction
  spline S1629 degree 3 poles (19.4112, 8.4923) (19.1644, 8.4923) (18.9643, 8.2923) (18.9643, 8.0455) knots 0 0 0 0 1 1 1 1
  line L5113 (19.4112, 8.4923) -> (19.1644, 8.4923) construction
  line L5114 (19.1644, 8.4923) -> (18.9643, 8.2923) construction
  line L5115 (18.9643, 8.2923) -> (18.9643, 8.0455) construction
  spline S1630 degree 3 poles (18.9643, 8.0455) (18.9643, 7.7987) (19.1644, 7.5984) (19.4112, 7.5984) knots 0 0 0 0 1 1 1 1
  line L5116 (18.9643, 8.0455) -> (18.9643, 7.7987) construction
  line L5117 (18.9643, 7.7987) -> (19.1644, 7.5984) construction
  line L5118 (19.1644, 7.5984) -> (19.4112, 7.5984) construction
  spline S1631 degree 3 poles (19.4112, 7.5984) (19.658, 7.5984) (19.8582, 7.7987) (19.8582, 8.0455) knots 0 0 0 0 1 1 1 1
  line L5119 (19.4112, 7.5984) -> (19.658, 7.5984) construction
  line L5120 (19.658, 7.5984) -> (19.8582, 7.7987) construction
  line L5121 (19.8582, 7.7987) -> (19.8582, 8.0455) construction
  spline S1632 degree 3 poles (19.8582, 10.5996) (19.8582, 10.8464) (19.658, 11.0465) (19.4112, 11.0465) knots 0 0 0 0 1 1 1 1
  line L5122 (19.8582, 10.5996) -> (19.8582, 10.8464) construction
  line L5123 (19.8582, 10.8464) -> (19.658, 11.0465) construction
  line L5124 (19.658, 11.0465) -> (19.4112, 11.0465) construction
  spline S1633 degree 3 poles (19.4112, 11.0465) (19.1644, 11.0465) (18.9643, 10.8464) (18.9643, 10.5996) knots 0 0 0 0 1 1 1 1
  line L5125 (19.4112, 11.0465) -> (19.1644, 11.0465) construction
  line L5126 (19.1644, 11.0465) -> (18.9643, 10.8464) construction
  line L5127 (18.9643, 10.8464) -> (18.9643, 10.5996) construction
  spline S1634 degree 3 poles (18.9643, 10.5996) (18.9643, 10.3528) (19.1644, 10.1525) (19.4112, 10.1525) knots 0 0 0 0 1 1 1 1
  line L5128 (18.9643, 10.5996) -> (18.9643, 10.3528) construction
  line L5129 (18.9643, 10.3528) -> (19.1644, 10.1525) construction
  line L5130 (19.1644, 10.1525) -> (19.4112, 10.1525) construction
  spline S1635 degree 3 poles (19.4112, 10.1525) (19.658, 10.1525) (19.8582, 10.3528) (19.8582, 10.5996) knots 0 0 0 0 1 1 1 1
  line L5131 (19.4112, 10.1525) -> (19.658, 10.1525) construction
  line L5132 (19.658, 10.1525) -> (19.8582, 10.3528) construction
  line L5133 (19.8582, 10.3528) -> (19.8582, 10.5996) construction
  spline S1636 degree 3 poles (22.7955, 11.7489) (22.7955, 11.9957) (22.5952, 12.1959) (22.3485, 12.1959) knots 0 0 0 0 1 1 1 1
  line L5134 (22.7955, 11.7489) -> (22.7955, 11.9957) construction
  line L5135 (22.7955, 11.9957) -> (22.5952, 12.1959) construction
  line L5136 (22.5952, 12.1959) -> (22.3485, 12.1959) construction
  spline S1637 degree 3 poles (22.3485, 12.1959) (22.1017, 12.1959) (21.9014, 11.9957) (21.9014, 11.7489) knots 0 0 0 0 1 1 1 1
  line L5137 (22.3485, 12.1959) -> (22.1017, 12.1959) construction
  line L5138 (22.1017, 12.1959) -> (21.9014, 11.9957) construction
  line L5139 (21.9014, 11.9957) -> (21.9014, 11.7489) construction
  spline S1638 degree 3 poles (21.9014, 11.7489) (21.9014, 11.5021) (22.1017, 11.302) (22.3485, 11.302) knots 0 0 0 0 1 1 1 1
  line L5140 (21.9014, 11.7489) -> (21.9014, 11.5021) construction
  line L5141 (21.9014, 11.5021) -> (22.1017, 11.302) construction
  line L5142 (22.1017, 11.302) -> (22.3485, 11.302) construction
  spline S1639 degree 3 poles (22.3485, 11.302) (22.5952, 11.302) (22.7955, 11.5021) (22.7955, 11.7489) knots 0 0 0 0 1 1 1 1
  line L5143 (22.3485, 11.302) -> (22.5952, 11.302) construction
  line L5144 (22.5952, 11.302) -> (22.7955, 11.5021) construction
  line L5145 (22.7955, 11.5021) -> (22.7955, 11.7489) construction
  spline S1640 degree 3 poles (25.3496, 11.7489) (25.3496, 11.9957) (25.1494, 12.1959) (24.9026, 12.1959) knots 0 0 0 0 1 1 1 1
  line L5146 (25.3496, 11.7489) -> (25.3496, 11.9957) construction
  line L5147 (25.3496, 11.9957) -> (25.1494, 12.1959) construction
  line L5148 (25.1494, 12.1959) -> (24.9026, 12.1959) construction
  spline S1641 degree 3 poles (24.9026, 12.1959) (24.6558, 12.1959) (24.4555, 11.9957) (24.4555, 11.7489) knots 0 0 0 0 1 1 1 1
  line L5149 (24.9026, 12.1959) -> (24.6558, 12.1959) construction
  line L5150 (24.6558, 12.1959) -> (24.4555, 11.9957) construction
  line L5151 (24.4555, 11.9957) -> (24.4555, 11.7489) construction
  spline S1642 degree 3 poles (24.4555, 11.7489) (24.4555, 11.5021) (24.6558, 11.302) (24.9026, 11.302) knots 0 0 0 0 1 1 1 1
  line L5152 (24.4555, 11.7489) -> (24.4555, 11.5021) construction
  line L5153 (24.4555, 11.5021) -> (24.6558, 11.302) construction
  line L5154 (24.6558, 11.302) -> (24.9026, 11.302) construction
  spline S1643 degree 3 poles (24.9026, 11.302) (25.1494, 11.302) (25.3496, 11.5021) (25.3496, 11.7489) knots 0 0 0 0 1 1 1 1
  line L5155 (24.9026, 11.302) -> (25.1494, 11.302) construction
  line L5156 (25.1494, 11.302) -> (25.3496, 11.5021) construction
  line L5157 (25.3496, 11.5021) -> (25.3496, 11.7489) construction
  spline S1644 degree 3 poles (22.7955, 14.303) (22.7955, 14.5498) (22.5952, 14.75) (22.3485, 14.75) knots 0 0 0 0 1 1 1 1
  line L5158 (22.7955, 14.303) -> (22.7955, 14.5498) construction
  line L5159 (22.7955, 14.5498) -> (22.5952, 14.75) construction
  line L5160 (22.5952, 14.75) -> (22.3485, 14.75) construction
  spline S1645 degree 3 poles (22.3485, 14.75) (22.1017, 14.75) (21.9014, 14.5498) (21.9014, 14.303) knots 0 0 0 0 1 1 1 1
  line L5161 (22.3485, 14.75) -> (22.1017, 14.75) construction
  line L5162 (22.1017, 14.75) -> (21.9014, 14.5498) construction
  line L5163 (21.9014, 14.5498) -> (21.9014, 14.303) construction
  spline S1646 degree 3 poles (21.9014, 14.303) (21.9014, 14.0562) (22.1017, 13.8561) (22.3485, 13.8561) knots 0 0 0 0 1 1 1 1
  line L5164 (21.9014, 14.303) -> (21.9014, 14.0562) construction
  line L5165 (21.9014, 14.0562) -> (22.1017, 13.8561) construction
  line L5166 (22.1017, 13.8561) -> (22.3485, 13.8561) construction
  spline S1647 degree 3 poles (22.3485, 13.8561) (22.5952, 13.8561) (22.7955, 14.0562) (22.7955, 14.303) knots 0 0 0 0 1 1 1 1
  line L5167 (22.3485, 13.8561) -> (22.5952, 13.8561) construction
  line L5168 (22.5952, 13.8561) -> (22.7955, 14.0562) construction
  line L5169 (22.7955, 14.0562) -> (22.7955, 14.303) construction
  spline S1648 degree 3 poles (25.3496, 14.303) (25.3496, 14.5498) (25.1494, 14.75) (24.9026, 14.75) knots 0 0 0 0 1 1 1 1
  line L5170 (25.3496, 14.303) -> (25.3496, 14.5498) construction
  line L5171 (25.3496, 14.5498) -> (25.1494, 14.75) construction
  line L5172 (25.1494, 14.75) -> (24.9026, 14.75) construction
  spline S1649 degree 3 poles (24.9026, 14.75) (24.6558, 14.75) (24.4555, 14.5498) (24.4555, 14.303) knots 0 0 0 0 1 1 1 1
  line L5173 (24.9026, 14.75) -> (24.6558, 14.75) construction
  line L5174 (24.6558, 14.75) -> (24.4555, 14.5498) construction
  line L5175 (24.4555, 14.5498) -> (24.4555, 14.303) construction
  spline S1650 degree 3 poles (24.4555, 14.303) (24.4555, 14.0562) (24.6558, 13.8561) (24.9026, 13.8561) knots 0 0 0 0 1 1 1 1
  line L5176 (24.4555, 14.303) -> (24.4555, 14.0562) construction
  line L5177 (24.4555, 14.0562) -> (24.6558, 13.8561) construction
  line L5178 (24.6558, 13.8561) -> (24.9026, 13.8561) construction
  spline S1651 degree 3 poles (24.9026, 13.8561) (25.1494, 13.8561) (25.3496, 14.0562) (25.3496, 14.303) knots 0 0 0 0 1 1 1 1
  line L5179 (24.9026, 13.8561) -> (25.1494, 13.8561) construction
  line L5180 (25.1494, 13.8561) -> (25.3496, 14.0562) construction
  line L5181 (25.3496, 14.0562) -> (25.3496, 14.303) construction
  spline S1652 degree 3 poles (17.3041, 5.4914) (17.3041, 5.7382) (17.1039, 5.9382) (16.8571, 5.9382) knots 0 0 0 0 1 1 1 1
  line L5182 (17.3041, 5.4914) -> (17.3041, 5.7382) construction
  line L5183 (17.3041, 5.7382) -> (17.1039, 5.9382) construction
  line L5184 (17.1039, 5.9382) -> (16.8571, 5.9382) construction
  spline S1653 degree 3 poles (16.8571, 5.9382) (16.6103, 5.9382) (16.4102, 5.7382) (16.4102, 5.4914) knots 0 0 0 0 1 1 1 1
  line L5185 (16.8571, 5.9382) -> (16.6103, 5.9382) construction
  line L5186 (16.6103, 5.9382) -> (16.4102, 5.7382) construction
  line L5187 (16.4102, 5.7382) -> (16.4102, 5.4914) construction
  spline S1654 degree 3 poles (16.4102, 5.4914) (16.4102, 5.2446) (16.6103, 5.0443) (16.8571, 5.0443) knots 0 0 0 0 1 1 1 1
  line L5188 (16.4102, 5.4914) -> (16.4102, 5.2446) construction
  line L5189 (16.4102, 5.2446) -> (16.6103, 5.0443) construction
  line L5190 (16.6103, 5.0443) -> (16.8571, 5.0443) construction
  spline S1655 degree 3 poles (16.8571, 5.0443) (17.1039, 5.0443) (17.3041, 5.2446) (17.3041, 5.4914) knots 0 0 0 0 1 1 1 1
  line L5191 (16.8571, 5.0443) -> (17.1039, 5.0443) construction
  line L5192 (17.1039, 5.0443) -> (17.3041, 5.2446) construction
  line L5193 (17.3041, 5.2446) -> (17.3041, 5.4914) construction
  spline S1656 degree 3 poles (14.75, 5.4914) (14.75, 5.7382) (14.5498, 5.9382) (14.303, 5.9382) knots 0 0 0 0 1 1 1 1
  line L5194 (14.75, 5.4914) -> (14.75, 5.7382) construction
  line L5195 (14.75, 5.7382) -> (14.5498, 5.9382) construction
  line L5196 (14.5498, 5.9382) -> (14.303, 5.9382) construction
  spline S1657 degree 3 poles (14.303, 5.9382) (14.0562, 5.9382) (13.8561, 5.7382) (13.8561, 5.4914) knots 0 0 0 0 1 1 1 1
  line L5197 (14.303, 5.9382) -> (14.0562, 5.9382) construction
  line L5198 (14.0562, 5.9382) -> (13.8561, 5.7382) construction
  line L5199 (13.8561, 5.7382) -> (13.8561, 5.4914) construction
  spline S1658 degree 3 poles (13.8561, 5.4914) (13.8561, 5.2446) (14.0562, 5.0443) (14.303, 5.0443) knots 0 0 0 0 1 1 1 1
  line L5200 (13.8561, 5.4914) -> (13.8561, 5.2446) construction
  line L5201 (13.8561, 5.2446) -> (14.0562, 5.0443) construction
  line L5202 (14.0562, 5.0443) -> (14.303, 5.0443) construction
  spline S1659 degree 3 poles (14.303, 5.0443) (14.5498, 5.0443) (14.75, 5.2446) (14.75, 5.4914) knots 0 0 0 0 1 1 1 1
  line L5203 (14.303, 5.0443) -> (14.5498, 5.0443) construction
  line L5204 (14.5498, 5.0443) -> (14.75, 5.2446) construction
  line L5205 (14.75, 5.2446) -> (14.75, 5.4914) construction
  spline S1660 degree 3 poles (17.3041, 8.0455) (17.3041, 8.2923) (17.1039, 8.4923) (16.8571, 8.4923) knots 0 0 0 0 1 1 1 1
  line L5206 (17.3041, 8.0455) -> (17.3041, 8.2923) construction
  line L5207 (17.3041, 8.2923) -> (17.1039, 8.4923) construction
  line L5208 (17.1039, 8.4923) -> (16.8571, 8.4923) construction
  spline S1661 degree 3 poles (16.8571, 8.4923) (16.6103, 8.4923) (16.4102, 8.2923) (16.4102, 8.0455) knots 0 0 0 0 1 1 1 1
  line L5209 (16.8571, 8.4923) -> (16.6103, 8.4923) construction
  line L5210 (16.6103, 8.4923) -> (16.4102, 8.2923) construction
  line L5211 (16.4102, 8.2923) -> (16.4102, 8.0455) construction
  spline S1662 degree 3 poles (16.4102, 8.0455) (16.4102, 7.7987) (16.6103, 7.5984) (16.8571, 7.5984) knots 0 0 0 0 1 1 1 1
  line L5212 (16.4102, 8.0455) -> (16.4102, 7.7987) construction
  line L5213 (16.4102, 7.7987) -> (16.6103, 7.5984) construction
  line L5214 (16.6103, 7.5984) -> (16.8571, 7.5984) construction
  spline S1663 degree 3 poles (16.8571, 7.5984) (17.1039, 7.5984) (17.3041, 7.7987) (17.3041, 8.0455) knots 0 0 0 0 1 1 1 1
  line L5215 (16.8571, 7.5984) -> (17.1039, 7.5984) construction
  line L5216 (17.1039, 7.5984) -> (17.3041, 7.7987) construction
  line L5217 (17.3041, 7.7987) -> (17.3041, 8.0455) construction
  spline S1664 degree 3 poles (17.3041, 10.5996) (17.3041, 10.8464) (17.1039, 11.0465) (16.8571, 11.0465) knots 0 0 0 0 1 1 1 1
  line L5218 (17.3041, 10.5996) -> (17.3041, 10.8464) construction
  line L5219 (17.3041, 10.8464) -> (17.1039, 11.0465) construction
  line L5220 (17.1039, 11.0465) -> (16.8571, 11.0465) construction
  spline S1665 degree 3 poles (16.8571, 11.0465) (16.6103, 11.0465) (16.4102, 10.8464) (16.4102, 10.5996) knots 0 0 0 0 1 1 1 1
  line L5221 (16.8571, 11.0465) -> (16.6103, 11.0465) construction
  line L5222 (16.6103, 11.0465) -> (16.4102, 10.8464) construction
  line L5223 (16.4102, 10.8464) -> (16.4102, 10.5996) construction
  spline S1666 degree 3 poles (16.4102, 10.5996) (16.4102, 10.3528) (16.6103, 10.1525) (16.8571, 10.1525) knots 0 0 0 0 1 1 1 1
  line L5224 (16.4102, 10.5996) -> (16.4102, 10.3528) construction
  line L5225 (16.4102, 10.3528) -> (16.6103, 10.1525) construction
  line L5226 (16.6103, 10.1525) -> (16.8571, 10.1525) construction
  spline S1667 degree 3 poles (16.8571, 10.1525) (17.1039, 10.1525) (17.3041, 10.3528) (17.3041, 10.5996) knots 0 0 0 0 1 1 1 1
  line L5227 (16.8571, 10.1525) -> (17.1039, 10.1525) construction
  line L5228 (17.1039, 10.1525) -> (17.3041, 10.3528) construction
  line L5229 (17.3041, 10.3528) -> (17.3041, 10.5996) construction
  spline S1668 degree 3 poles (17.3041, 13.1537) (17.3041, 13.4005) (17.1039, 13.6006) (16.8571, 13.6006) knots 0 0 0 0 1 1 1 1
  line L5230 (17.3041, 13.1537) -> (17.3041, 13.4005) construction
  line L5231 (17.3041, 13.4005) -> (17.1039, 13.6006) construction
  line L5232 (17.1039, 13.6006) -> (16.8571, 13.6006) construction
  spline S1669 degree 3 poles (16.8571, 13.6006) (16.6103, 13.6006) (16.4102, 13.4005) (16.4102, 13.1537) knots 0 0 0 0 1 1 1 1
  line L5233 (16.8571, 13.6006) -> (16.6103, 13.6006) construction
  line L5234 (16.6103, 13.6006) -> (16.4102, 13.4005) construction
  line L5235 (16.4102, 13.4005) -> (16.4102, 13.1537) construction
  spline S1670 degree 3 poles (16.4102, 13.1537) (16.4102, 12.9069) (16.6103, 12.7067) (16.8571, 12.7067) knots 0 0 0 0 1 1 1 1
  line L5236 (16.4102, 13.1537) -> (16.4102, 12.9069) construction
  line L5237 (16.4102, 12.9069) -> (16.6103, 12.7067) construction
  line L5238 (16.6103, 12.7067) -> (16.8571, 12.7067) construction
  spline S1671 degree 3 poles (16.8571, 12.7067) (17.1039, 12.7067) (17.3041, 12.9069) (17.3041, 13.1537) knots 0 0 0 0 1 1 1 1
  line L5239 (16.8571, 12.7067) -> (17.1039, 12.7067) construction
  line L5240 (17.1039, 12.7067) -> (17.3041, 12.9069) construction
  line L5241 (17.3041, 12.9069) -> (17.3041, 13.1537) construction
  spline S1672 degree 3 poles (17.3041, 15.7078) (17.3041, 15.9546) (17.1039, 16.1547) (16.8571, 16.1547) knots 0 0 0 0 1 1 1 1
  line L5242 (17.3041, 15.7078) -> (17.3041, 15.9546) construction
  line L5243 (17.3041, 15.9546) -> (17.1039, 16.1547) construction
  line L5244 (17.1039, 16.1547) -> (16.8571, 16.1547) construction